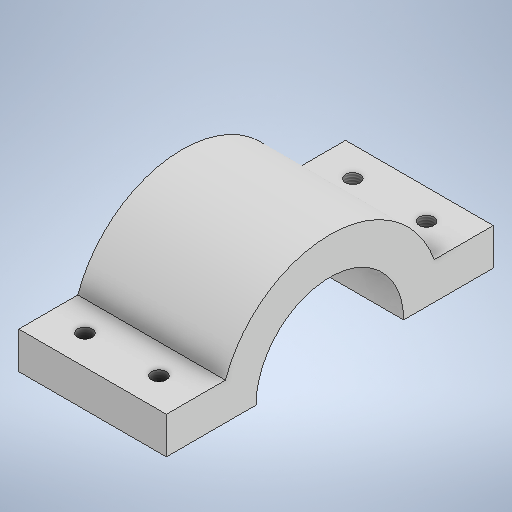
# Autodesk Inventor part: U_bracket
Saved by Autodesk Inventor 2025.3 (Build 293356030, 356C)
## iProperties
Created: 2026-06-25
Part Number: U_bracket
Material: Generic
Document SubType Name: Modeling
Designer: user
Density: 1 g/cm^3
Appearance: Default
Author: user
Autodesk Inventor part; units mm, degrees
ref_plane "YZ Plane" through (0, 0, 0) normal (1, 0, 0) x (0, 1, 0)
ref_plane "XZ Plane" through (0, 0, 0) normal (0, 1, 0) x (-1, 0, 0)
ref_plane "XY Plane" through (0, 0, 0) normal (0, 0, 1) x (1, 0, 0)
sketch "Sketch1" plane through (0, 0, 0) normal (1, 0, 0) x (0, 1, 0)
  arc A0 (0, -20) -> (0, 20) centre (0, 0) ccw
  arc A1 (10, -28.2843) -> (10, 28.2843) centre (0, 0) ccw
  line L0 (10, 44.2843) -> (0, 44.2843)
  line L1 (0, -44.2843) -> (10, -44.2843)
  line L2 (10, -44.2843) -> (10, -28.2843)
  line L3 (10, 28.2843) -> (10, 44.2843)
  line L4 (0, 44.2843) -> (0, 20)
  line L5 (0, -20) -> (0, -44.2843)
  line L6 (0, 44.2843) -> (0, 20)
  line L7 (0, -20) -> (0, -44.2843)
  dimension "d2" = 30
  dimension "d3" = 20
  dimension "d5" = 10
  dimension "d6" = 10
  dimension "d11" = 16
  dimension "d12" = 16
  constraints: 16 end point, 5 parallel, 4 point on circle, 2 centre point, 2 coincident, 2 perpendicular, 2 vertical, 1 horizontal
  measures "d2" radius of A1
  measures "d3" radius of A0
  measures "d5" distance from line of L3 point (0, 0)
  measures "d6" distance from line of point (0, 0) L2
  measures "d11" distance of L3.start L0.start
  measures "d12" distance of L1.end L2.end
extrude "Extrusion1" add sketch "Sketch1" along normal blind 40
sketch "Sketch4" plane through (0, 10, 44.2843) normal (0, 1, 0) x (1, 0, 0)
  line L0 (0, 0) -> (0, 24.2843) construction
  line L1 (0, 8) -> (0, -32) construction
  line L2 (0, 8) -> (40.1355, 8) construction
  line L3 (0, 0) -> (40, 0) projected
  line L4 (10, 0) -> (-6, 0)
  line L5 (10, 0) -> (10, 16.0426) construction
  line L6 (30, 0) -> (30, 16) construction
  line L7 (0, 16) -> (40, 16) projected
  point P0 (0, 44.2843)
  dimension "d13" = 40
  dimension "d14" = 16
  constraints: 10 end point, 4 point on line, 2 collinear, 1 vertical
  measures "d13" distance of L1.start L1.end
  measures "d14" distance of L4.start L4.end
sketch "Sketch5" plane through (0, 10, 44.2843) normal (0, 1, 0) x (1, 0, 0)
  point P0 (0, 44.2843)
  point P1 (9.9387, 7.9868)
  point P2 (29.9524, 8.0308)
hole "Hole1" at (9.9387, 10, 36.2975) at (29.9524, 10, 36.2535) direction (0, -1, 0) diameter 4 end through all
thread "Thread1" size "M4x0.7" class "6H" standard "ANSI Metric M Profile" length 150
thread "Thread2" size "M4x0.7" class "6H" standard "ANSI Metric M Profile" length 150
mirror "Mirror1" about plane through (0, 0, 0) normal (0, 0, 1) of "Hole1"
thread "Thread3" size "M4x0.7" class "6H" standard "ANSI Metric M Profile" length 150
thread "Thread4" size "M4x0.7" class "6H" standard "ANSI Metric M Profile" length 150
body "Solid1"
